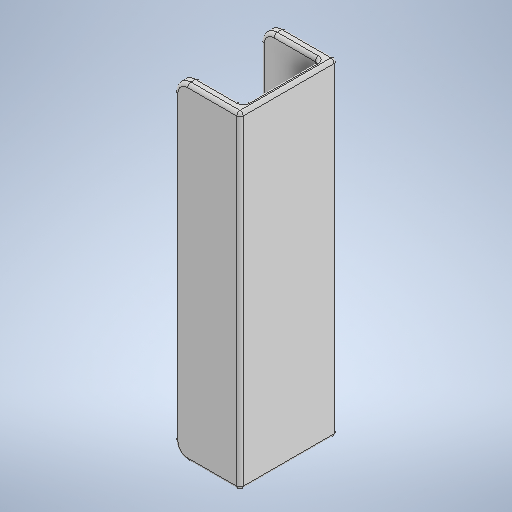
# Autodesk Inventor part: Соединитель
Saved by Autodesk Inventor 2025 (Build 290162000, 162)
## iProperties
Created: 2025-05-20
Part Number: Соединитель
Material: Типовые
Document SubType Name: Modeling
Designer: vinogradov
Density: 1 g/cm^3
Appearance: По умолчанию
Author: vinogradov
Autodesk Inventor part; units mm, degrees
ref_plane "YZ Plane" through (0, 0, 0) normal (1, 0, 0) x (0, 1, 0)
ref_plane "XZ Plane" through (0, 0, 0) normal (0, 1, 0) x (-1, 0, 0)
ref_plane "XY Plane" through (0, 0, 0) normal (0, 0, 1) x (1, 0, 0)
sketch "Эскиз2" plane through (0, 0, 0) normal (0, 1, 0) x (-1, 0, 0)
  line L0 (0, 0) -> (10, 0)
  line L1 (10, 0) -> (10, -1.7)
  line L2 (10, -1.7) -> (1.2, -1.7)
  line L3 (1.2, -1.7) -> (1.2, -13.2)
  line L4 (1.2, -13.2) -> (10, -13.2)
  line L5 (10, -13.2) -> (10, -14.9)
  line L6 (10, -14.9) -> (0, -14.9)
  line L7 (0, -14.9) -> (0, 0)
  dimension "d0" = 10
  dimension "d1" = 1.7
  dimension "d4" = 1.7
  dimension "d5" = 1.2
  dimension "d10" = 14.9
  constraints: 16 end point, 6 perpendicular, 2 point on line, 1 horizontal
  measures "d0" distance of L0.start L0.end
  measures "d1" distance of L0.end L1.end
  measures "d4" distance of L4.end L5.end
  measures "d5" distance between parallel lines of L7 L3
  measures "d10" distance between parallel lines of L6 L0
extrude "Выдавливание1" add sketch "Эскиз2" along normal blind 50
fillet "Сопряжение1" radius 2 4 edges at (-10, 50, -14.05) (-10, 50, -0.85) (-10, 0, -14.05) (-10, 0, -0.85)
fillet "Сопряжение2" radius 0.5 28 edges at (0, 25, -14.9) (-9.4142, 49.4142, -14.9) (-10, 25, -14.9) (-9.4142, 0.5858, -14.9) (-4, 0, -14.9) (-4, 50, -14.9) (-9.4142, 49.4142, -13.2) (-10, 25, -13.2) (-9.4142, 0.5858, -13.2) (-4.6, 0, -13.2) (-4.6, 50, -13.2) (-1.2, 50, -7.45) (0, 50, -7.45) (-9.4142, 49.4142, 0) (-10, 25, 0) (-9.4142, 0.5858, 0) (-4, 0, 0) (-4, 50, 0) (-9.4142, 49.4142, -1.7) (-10, 25, -1.7) (-9.4142, 0.5858, -1.7) (-4.6, 0, -1.7) (-4.6, 50, -1.7) (-1.2, 25, -1.7) (-1.2, 0, -7.45) (0, 0, -7.45) (-1.2, 25, -13.2) (0, 25, 0)
